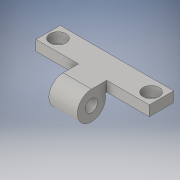
# Autodesk Inventor part: camera holderpt2
Saved by Autodesk Inventor 2016 (Build 200138000, 138)
## iProperties
Created: 2015-10-02
Part Number: camera holderpt2
Material: Generic
Document SubType Name: Modeling
Designer: Zachary
Density: 1 g/cm^3
Appearance: Default
Author: Zachary
Autodesk Inventor part; units mm, degrees
ref_plane "YZ Plane" through (0, 0, 0) normal (1, 0, 0) x (0, 1, 0)
ref_plane "XZ Plane" through (0, 0, 0) normal (0, 1, 0) x (-1, 0, 0)
ref_plane "XY Plane" through (0, 0, 0) normal (0, 0, 1) x (1, 0, 0)
sketch "Sketch1" plane through (0, 0, 0) normal (0, 1, 0) x (-1, 0, 0)
  line L0 (0, 0) -> (28, 0)
  line L1 (28, 0) -> (28, -6)
  line L2 (28, -6) -> (0, -6)
  line L3 (0, -6) -> (0, 0)
  dimension "d0" = 28
  dimension "d1" = 6
  constraints: 8 end point, 2 parallel, 1 horizontal, 1 perpendicular
  measures "d0" distance of L1.end L2.end
  measures "d1" distance of L0.end L1.end
extrude "Extrusion1" add sketch "Sketch1" along normal blind 2.54
hole "Hole1" at (-25.5, 2.54, -2.952) direction (0, -1, 0) diameter 4 end through all
hole "Hole2" at (-2.5, 2.54, -2.952) direction (0, -1, 0) diameter 4 end through all
sketch "Sketch2" plane through (0, 0, 0) normal (1, 0, 0) x (0, 0, -1)
  circle A0 centre (-3.7852, -0.96) radius 3.5
  line L0 (-3.7852, 2.54) -> (0.6598, 2.54)
  line L1 (0, 2.54) -> (6, 2.54) projected
  line L2 (6, 0) -> (0, 0) projected
  line L3 (-0.4194, 0) -> (0, 0)
  line L4 (0, 0) -> (-0.4194, 0)
  line L5 (0.2994, 0) -> (-3.7852, 0)
  line L6 (-3.7852, 0) -> (-3.7852, 2.54)
  line L7 (-3.7852, 2.54) -> (0.2994, 2.54)
  line L8 (0.2994, 2.54) -> (0.2994, 0)
  line L9 (0.2994, 2.54) -> (-3.6886, 2.54)
  line L10 (-3.6886, 2.54) -> (-3.6886, 0)
  line L11 (-3.6886, 0) -> (0.2994, 0)
  line L12 (0.2994, 0) -> (0.2994, 2.54)
  dimension "d22" = 7
  dimension "d41" = 4.445
  constraints: 22 end point, 5 equal length, 3 horizontal, 3 point on line, 2 perpendicular, 2 point on circle, 1 centre point
  measures "d22" diameter of A0
  measures "d41" distance of L0.start L0.end
extrude "Extrusion2" add sketch "Sketch2" against normal blind 28
sketch "Sketch3" plane through (0, 2.54, 0) normal (0, 1, 0) x (1, 0, 0)
  line L0 (-28, 0) -> (-17.5, 0)
  line L1 (-17.5, 0) -> (-17.5, -12.7)
  line L2 (-17.5, -12.7) -> (-28, -12.7)
  line L3 (-28, -12.7) -> (-28, 0)
  line L4 (0, 0) -> (0, 6) projected
  line L5 (0, 0) -> (-10.5, 0)
  line L6 (-10.5, 0) -> (-10.5, -9.3969)
  line L7 (-10.5, -9.3969) -> (0, -9.3969)
  line L8 (0, -9.3969) -> (0, 0)
  dimension "d28" = 7
  dimension "d29" = 10.5
  dimension "d42" = 12.7
  constraints: 16 end point, 4 parallel, 2 horizontal, 2 perpendicular
  measures "d28" distance between parallel lines of L6 L1
  measures "d29" distance of L1.end L2.end
  measures "d42" distance of L2.end L0.start
extrude "Extrusion3" cut sketch "Sketch3" against normal blind 28
hole "Hole3" at (-10.5, -0.96, 3.7852) direction (-1, 0, 0) diameter 3 end through all
body "Solid1"
